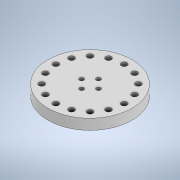
# Autodesk Inventor part: dischetto
Saved by Autodesk Inventor 2020.2 (Build 242310000, 310)
## iProperties
Created: 2020-02-12
Part Number: dischetto
Material: Generico
Document SubType Name: Modeling
Designer: socci
Density: 1 g/cm^3
Appearance: Default
Author: socci
Autodesk Inventor part; units mm, degrees
ref_plane "YZ Plane" through (0, 0, 0) normal (1, 0, 0) x (0, 1, 0)
ref_plane "XZ Plane" through (0, 0, 0) normal (0, 1, 0) x (-1, 0, 0)
ref_plane "XY Plane" through (0, 0, 0) normal (0, 0, 1) x (1, 0, 0)
sketch "Schizzo1" plane through (0, 0, 0) normal (0, 1, 0) x (-1, 0, 0)
  circle A0 centre (0, 0) radius 40
  dimension "d0" = 80
  constraints: 1 centre point, 1 coincident
  measures "d0" diameter of A0
extrude "Estrusione1" add sketch "Schizzo1" along normal blind 10
sketch "Schizzo2" plane through (0, 10, 0) normal (0, 1, 0) x (1, 0, 0)
  line L0 (0, -8) -> (0, 8)
  line L1 (0, -8) -> (16, -8) construction
  line L2 (-8, 0) -> (8, 0)
  line L3 (-8, 0) -> (8, 0) construction
  point P0 (0, 0)
  point P1 (0, 0)
  dimension "d4" = 16
  dimension "d5" = 90
  dimension "d6" = 16
  dimension "d7" = 0
  constraints: 8 end point, 3 horizontal, 2 equal length, 2 midpoint, 1 coincident, 1 vertical
  measures "d4" distance of L0.start L0.end
  measures "d5" angle of L1 L0
  measures "d6" distance of L2.start L2.end
  measures "d7" distance between parallel lines of L2 L3
hole "Foro1" at (-8, 10, 0) at (0, 10, 8) at (8, 10, 0) at (0, 10, -8) direction (0, -1, 0) diameter 4.2 depth 8.8 tip angle 118
sketch "Schizzo3" plane through (0, 10, 0) normal (0, 1, 0) x (1, 0, 0)
  line L0 (0, 0) -> (0, 32.5)
  point P0 (-12.4372, 30.0261)
  point P1 (-22.981, 22.981)
  point P2 (-30.0261, 12.4372)
  point P3 (-32.5, 0)
  point P4 (-30.0261, -12.4372)
  point P5 (-22.981, -22.981)
  point P6 (-12.4372, -30.0261)
  point P7 (0, -32.5)
  point P8 (12.4372, -30.0261)
  point P9 (22.981, -22.981)
  point P10 (30.0261, -12.4372)
  point P11 (32.5, 0)
  point P12 (30.0261, 12.4372)
  point P13 (22.981, 22.981)
  point P14 (12.4372, 30.0261)
  point P15 (24.3182, -23.5879)
  dimension "d15" = 32.5
  dimension "d19" = 360
  constraints: 2 end point, 1 coincident, 1 vertical, 17 other
  measures "d15" distance of L0.start L0.end
hole "Foro2" at (0, 10, -32.5) at (-30.0261, 10, 12.4372) at (-32.5, 10, 0) at (-30.0261, 10, -12.4372) at (-22.981, 10, -22.981) at (-12.4372, 10, -30.0261) at (0, 10, -32.5) at (12.4372, 10, -30.0261) at (22.981, 10, -22.981) at (30.0261, 10, -12.4372) at (32.5, 10, 0) at (30.0261, 10, 12.4372) at (22.981, 10, 22.981) at (12.4372, 10, 30.0261) at (0, 10, 32.5) at (-12.4372, 10, 30.0261) at (-22.981, 10, 22.981) direction (0, -1, 0) diameter 5.5 depth 8.8 tip angle 118 clearance for "Vite a testa svasata piana ISO 2009/7046" size "M5" standard "ISO"
